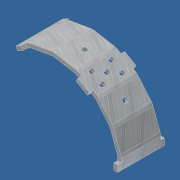
# Autodesk Inventor part: Lateral Wheel Casing 1764
Saved by Autodesk Inventor 2011 (Build 150239000, 239)
## iProperties
Created: 2010-01-13
Part Number: Lateral Wheel Casing 1764
Document SubType Name: Modeling
Designer: wbridges
Density: 1 g/cm^3
Author: wbridges
Autodesk Inventor part; units mm, degrees
ref_plane "YZ Plane" through (0, 0, 0) normal (1, 0, 0) x (0, 1, 0)
ref_plane "XZ Plane" through (0, 0, 0) normal (0, 1, 0) x (-1, 0, 0)
ref_plane "XY Plane" through (0, 0, 0) normal (0, 0, 1) x (1, 0, 0)
sketch "Sketch1" plane through (0, 0, 0) normal (0, 0, 1) x (1, 0, 0)
  line L0 (0, 0) -> (-2.413, 0)
  line L1 (-2.413, 0) -> (-2.413, 7.4633)
  line L2 (-2.413, 7.4633) -> (0, 7.4633)
  line L3 (0, 7.4633) -> (0, 0)
  line L4 (0, 7.4633) -> (-5.2908, 21.8786)
  line L5 (-2.413, 7.0345) -> (-7.5561, 21.0472)
  line L6 (-5.2908, 21.8786) -> (-7.5561, 21.0472)
  line L7 (-5.2908, 21.8786) -> (-15.1283, 33.6567)
  line L8 (-7.4116, 20.6536) -> (-16.9803, 32.1099)
  line L9 (-15.1283, 33.6567) -> (-16.9803, 32.1099)
  line L10 (-15.1283, 33.6567) -> (-21.9626, 37.6026)
  line L11 (-21.9626, 37.6026) -> (-23.1691, 35.5128)
  line L12 (-23.1691, 35.5128) -> (-16.7057, 31.7812)
  line L13 (-18.2781, 35.4753) -> (-19.4846, 33.3856)
  line L14 (-2.413, 0) -> (0, 0)
  line L15 (0, 0) -> (0, 4.2545)
  line L16 (0, 4.2545) -> (-2.413, 4.2545)
  line L17 (-2.413, 4.2545) -> (-2.413, 0)
  line L18 (-23.1691, 35.5128) -> (-29.6326, 39.2445)
  line L19 (-29.6326, 39.2445) -> (-16.7057, 31.7812)
  circle A0 centre (-43.688, -0.3009) radius 41.275
  dimension "d2" = 2.413
  dimension "d8" = 2.413
  dimension "d9" = 2.413
  dimension "d10" = 2.413
  dimension "d23" = 4.2545
  dimension "d24" = 4.2545
  dimension "d41" = 82.55
  dimension "d44" = 60
  constraints: 40 end point, 7 parallel, 7 perpendicular, 6 point on line, 4 equal length, 4 tangent, 2 horizontal, 1 centre point, 1 collinear
  measures "d2" distance of L0.start L0.end
  measures "d8" distance between parallel lines of L4 L5
  measures "d9" distance between parallel lines of L8 L7
  measures "d10" distance between parallel lines of L10 L12
  measures "d23" distance between parallel lines of L11 L13
  measures "d24" distance between parallel lines of L0 L16
  measures "d41" diameter of A0
  measures "d44" angle of L14 L11
extrude "Extrusion1" add sketch "Sketch1" against normal blind 12.7 contours L0 L1 L16 L3 | L11 L10 L13 L12 | L16 L1 L2 L3 | L5 L6 L4 L2 L1 | L8 L9 L7 L6 L5 | L13 L10 L9 L8 L12
extrude "Extrusion2" add sketch "Sketch1" along normal blind 2.413 contours L0 L1 L16 L3 | L11 L10 L13 L12
sketch "Sketch2" plane through (-15.1283, 33.6567, 0) normal (0.7675059, 0.6410419, 0) x (0, 0, -1)
  line L0 (12.7, -15.346) -> (12.7, 0) projected
  circle A0 centre (12.7, -7.673) radius 1.5875
  point P0 (0, -35.5296)
  dimension "d27" = 3.175
  constraints: 1 centre point, 1 midpoint
  measures "d27" diameter of A0
extrude "Extrusion3" cut sketch "Sketch2" against normal through all
sketch "Sketch3" plane through (-15.1283, 33.6567, 0) normal (0.5, 0.8660254, 0) x (0.8660254, -0.5, 0)
  line L0 (0, 12.7) -> (-7.8917, 12.7) projected
  line L1 (-7.8917, 12.7) -> (-7.8917, -2.413) projected
  circle A0 centre (-7.8917, 12.7) radius 1.5875
  circle A1 centre (-3.9229, 6.35) radius 1.5875
  point P0 (29.9298, 0)
  dimension "d30" = 3.175
  dimension "d31" = 0
  dimension "d32" = 3.175
  dimension "d33" = 6.35
  dimension "d34" = 3.9688
  constraints: 2 centre point, 1 point on line
  measures "d30" diameter of A0
  measures "d31" distance from line of L0 A0.centre
  measures "d32" diameter of A1
  measures "d33" distance from line of L0 A1.centre
  measures "d34" distance from line of L1 A1.centre
extrude "Extrusion4" cut sketch "Sketch3" along normal through all both and the other way through all
fillet "Fillet1" radius 6.35 3 edges at (0, 7.4633, -6.35) (-5.2908, 21.8786, -6.35) (-15.1283, 33.6567, -6.35)
fillet "Fillet1" radius 3.175 3 edges at (-2.413, 7.0345, -6.35) (-7.4116, 20.6536, -6.35) (-16.7057, 31.7812, -6.35)
mirror "Mirror5" about plane through (-21.9626, 37.6026, 0) normal (-0.8660254, 0.5, 0) of "Extrusion2", "Extrusion1", "Extrusion3", "Extrusion4", "Fillet1"
mirror "Mirror6" about plane through (-19.1932, 34.6222, -12.7) normal (0, 0, -1) of "Extrusion2", "Extrusion1", "Extrusion3", "Extrusion4", "Fillet1", "Mirror5"
body "Solid1"
